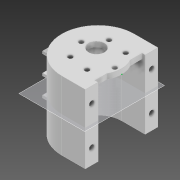
# Autodesk Inventor part: Motor_mount_Right
Saved by Autodesk Inventor 2020 (Build 240168000, 168)
## iProperties
Created: 2022-08-06
Part Number: Motor_mount_Right
Material: Generic
Document SubType Name: Modeling
Designer: umair_maher
Density: 1 g/cm^3
Appearance: Default
Author: umair_maher
Autodesk Inventor part; units mm, degrees
ref_plane "YZ Plane" through (0, 0, 0) normal (1, 0, 0) x (0, 1, 0)
ref_plane "XZ Plane" through (0, 0, 0) normal (0, 1, 0) x (-1, 0, 0)
ref_plane "XY Plane" through (0, 0, 0) normal (0, 0, 1) x (1, 0, 0)
sketch "Sketch1" plane through (0, 0, 0) normal (0, 1, 0) x (-1, 0, 0)
  circle A0 centre (0, 0) radius 18.5
  line L0 (5.5131, -10.5135) -> (5.5131, 1.8865)
  circle A1 centre (5.5131, -4.3135) radius 6.2
  line L1 (0, 0) -> (-24.4, 0)
  circle A2 centre (5.5131, -4.3135) radius 3
  circle A3 centre (5.5131, -4.3135) radius 40
  line L2 (-24.4, 0) -> (-24.4, -81.1676)
  line L3 (-24.4, -81.1676) -> (-24.4, 62.3764)
  line L4 (0, 0) -> (0, 28.5)
  line L5 (18.5, 0) -> (28.5, 0)
  line L6 (0, -18.5) -> (0, -28.5)
  arc A4 (28.5, 0) -> (0, 28.5) centre (0, 0) ccw
  arc A5 (0, -28.5) -> (28.5, 0) centre (0, 0) ccw
  line L7 (0, 18.5) -> (0, 23.5)
  line L8 (0, 18.5) -> (-18.5, 18.5)
  line L9 (-18.5, 18.5) -> (-18.5, 28.5)
  line L10 (-18.5, 28.5) -> (0, 28.5)
  line L11 (0, -18.5) -> (-18.5, -18.5)
  line L12 (-18.5, -18.5) -> (-18.5, -28.5)
  line L13 (-18.5, -28.5) -> (0, -28.5)
  line L14 (5.5131, -4.3135) -> (-72.1542, -4.3135)
  line L15 (0, 0) -> (5.5051, -4.3135)
  line L16 (0, 0) -> (6.9938, 0) construction
  line L17 (-16.0843, 18.5) -> (-16.0843, -18.5)
  circle A6 centre (0, 0) radius 15.5
  circle A7 centre (5.5051, -4.3135) radius 24.193
  circle A8 centre (5.5051, -4.3135) radius 10.066
  circle A9 centre (15.3445, -2.1897) radius 1.75
  circle A10 centre (9.5686, 12.1939) radius 1.75
  circle A11 centre (-5.7759, 14.3836) radius 1.75
  circle A12 centre (-15.3445, 2.1897) radius 1.75
  circle A13 centre (-9.5686, -12.1939) radius 1.75
  circle A14 centre (5.7759, -14.3836) radius 1.75
  point P0 (-17.3596, -28.5)
  point P1 (-18.5, -27.6751)
  point P2 (-17.3622, 28.5)
  point P3 (-18.5, 27.6767)
  point P4 (-16.0843, -9.1402)
  point P5 (-16.0843, 9.1402)
  dimension "d59" = 31
  dimension "d65" = 20.132
  dimension "d2" = 12.4
  dimension "d4" = 6
  dimension "d5" = 80
  dimension "d13" = 7
  dimension "d14" = 24.4
  dimension "d17" = 37
  dimension "d18" = 28.5
  dimension "d19" = 10
  dimension "d20" = 10
  dimension "d58" = 38.08
  dimension "d63" = 48.386
  dimension "d66" = 3.5
  dimension "d69" = 360
  constraints: 36 end point, 12 centre point, 8 point on line, 7 point on circle, 6 coincident, 5 perpendicular, 4 horizontal, 4 vertical, 2 concentric, 1 equal length, 1 midpoint, 1 parallel, 1 vertical alignment, 21 other
  measures "d2" distance of L0.start L0.end
  measures "d4" diameter of A2
  measures "d5" diameter of A3
  measures "d13" distance of point (5.513, -4.313) point (0, 0)
  measures "d14" distance from line of point (0, 0) L2
  measures "d17" diameter of A0
  measures "d18" distance of L1.start L4.end
  measures "d19" distance of L5.start L5.end
  measures "d20" distance of L6.start L6.end
  measures "d58" angle of L15 L16
  measures "d63" diameter of A7
  measures "d66" diameter of A9
extrude "Extrusion1" add sketch "Sketch1" along normal blind 4 contours A0 L17 L14 A6 A13 A14 A8 A9 A10 L4 | L5 A5 A7 L6 A0 | A0 L4 A7 A4 L5 | L4 A6 A11 A12 L17 A7 A0 | L8 A7 L4 | A0 A7 L8 | L11 A7 L17 A0 | L6 A7 L11 | A7 L17 A0 | A0 L17 L8 A7 | A6 A10 A9 A8 L4 | L4 A8 L1 A6 A12 A11 | A7 L8 L9 A3 L10 L4 | L4 A4 A7 | A0 L14 L17 | A7 A5 L6 | L6 L13 L12 L11 A7 | L11 L17 A7 | L17 A7 L1 A0 | L17 A12 L1 A7 | A8 A9 A6 A14 L14 A1 L15 L4 | L4 L1 A8 | A0 A7 L1 L17 L14 | L17 L1 A6 L14 | L1 A7 A0 | L15 A1 L14 A8 L1 | A8 L14 A6 L1 | L14 A8 A14 A6 A13 | L17 A12 A6 L1 | A3 L9 L10 | A9 A8 A14 A6
extrude "Extrusion2" add sketch "Sketch1" against normal blind 50 contours L5 A5 A7 L6 A0 | A0 L4 A7 A4 L5 | L8 A7 L4 | L6 A7 L11 | A7 L8 L9 A3 L10 L4 | L4 A4 A7 | A7 A5 L6 | L6 L13 L12 L11 A7 | A3 L9 L10
sketch "Sketch2" plane through (18.5, 4, 28.5) normal (1, 0, 0) x (0, 0, -1)
  point P0 (28.5, -4)
ref_plane "Work Plane1" through (0, -22, 0) normal (0, 1, 0) x (1, 0, 0)
sketch "Sketch5" plane through (0, -22, 0) normal (0, 1, 0) x (1, 0, 0)
  arc A0 (0, 28.5) -> (0, -28.5) centre (0, 0) ccw projected
  line L0 (-28.5, 0) -> (-28.5, -10)
  line L1 (-28.5, -10) -> (-28.5, 10)
  line L2 (-28.5, 10) -> (-23.5, 10)
  line L3 (-23.5, 10) -> (-23.5, -10)
  line L4 (-23.5, -10) -> (-28.5, -10)
  line L5 (-28.5, -10) -> (-33.5, -10)
  line L6 (-33.5, -10) -> (-33.5, 10)
  line L7 (-33.5, 10) -> (-28.5, 10)
  line L8 (-28.5, 10) -> (-28.5, 7)
  line L9 (-28.5, 7) -> (-29.5, 7)
  line L10 (-29.5, 7) -> (-32.5, 7)
  line L11 (-32.5, 7) -> (-33.5, 7)
  line L12 (-28.5, -10) -> (-28.5, -7)
  line L13 (-28.5, -7) -> (-29.5, -7)
  line L14 (-29.5, -7) -> (-32.5, -7)
  line L15 (-32.5, -7) -> (-33.5, -7)
  line L16 (-33.5, -7) -> (-33.5, 7)
  line L17 (-32.5, -7) -> (-32.5, 7)
  line L18 (-29.5, -7) -> (-29.5, 7)
  point P0 (0, 0)
  point P1 (-26.688, 10)
  point P2 (-26.688, -10)
  dimension "d31" = 10
  dimension "d32" = 20
  dimension "d33" = 5
  dimension "d34" = 5
  dimension "d35" = 3
  dimension "d36" = 1
  dimension "d37" = 3
  dimension "d38" = 3
  dimension "d39" = 1
  dimension "d40" = 3
  dimension "d41" = 1
  constraints: 38 end point, 10 point on line, 7 perpendicular, 1 collinear, 1 point on circle, 1 tangent, 1 vertical
  measures "d31" distance of L0.start L0.end
  measures "d32" distance of L0.end L1.end
  measures "d33" distance of L1.end L2.end
  measures "d34" distance of L0.end L5.end
  measures "d35" distance of L1.end L8.end
  measures "d36" distance of L8.end L9.end
  measures "d37" distance of L9.end L10.end
  measures "d38" distance of L0.end L12.end
  measures "d39" distance of L12.end L13.end
  measures "d40" distance of L13.end L14.end
  measures "d41" distance of L14.end L15.end
extrude "Extrusion3" add sketch "Sketch5" along normal blind 2 contours A0 L1 L2 | A0 L4 L0 | L0 L13 L18 L9 L1 | L1 L9 L10 L11 L6 L7 | L0 L5 L6 L15 L14 L13 | L11 L17 L15 L6
pattern_linear "Rectangular Pattern1" count 2 spacing 15 along (0, 1, 0) of "Extrusion3"
pattern_linear "Rectangular Pattern2" count 2 spacing 15 along (0, -1, 0) of "Extrusion3"
sketch "Sketch6" plane through (18.5, 4, 28.5) normal (1, 0, 0) x (0, 0, -1)
  line L0 (57, 0) -> (0, 0) projected
  line L1 (0, 0) -> (10, 0)
  line L2 (10, 0) -> (5, 0)
  line L3 (5, 0) -> (5, -54)
  line L4 (0, -54) -> (57, -54) projected
  line L5 (5, -27) -> (5, -12)
  line L6 (5, -12) -> (5, -42)
  circle A0 centre (5, -42) radius 2
  circle A1 centre (5, -12) radius 2
  point P0 (28.5, -4)
  dimension "d50" = 5
  dimension "d51" = 15
  dimension "d52" = 30
  dimension "d53" = 4
  dimension "d54" = 4
  constraints: 10 end point, 3 point on line, 2 centre point, 2 coincident, 2 midpoint, 1 horizontal, 1 perpendicular
  measures "d50" distance of L1.end L2.end
  measures "d51" distance of L5.start L5.end
  measures "d52" distance of L5.end L6.end
  measures "d53" diameter of A0
  measures "d54" diameter of A1
extrude "Extrusion4" cut sketch "Sketch6" against normal blind 15
mirror "Mirror1" about plane through (0, 0, 0) normal (0, 0, 1) of "Extrusion4"
sketch "Sketch7" plane through (18.5, 4, 28.5) normal (1, 0, 0) x (0, 0, -1)
  point P0 (28.5, -4)
body "Solid1"
